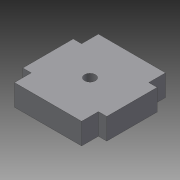
# Autodesk Inventor part: Frame_Upper_Plate_Pulley_A
Saved by Autodesk Inventor 2014 (Build 180170000, 170)
## iProperties
Created: 2014-08-25
Part Number: Frame_Upper_Plate_Pulley_A
Material: Generic
Document SubType Name: Modeling
Designer: ThatOtherGuy
Density: 1 g/cm^3
Appearance: Default
Author: ThatOtherGuy
Autodesk Inventor part; units mm, degrees
ref_plane "YZ Plane" through (0, 0, 0) normal (1, 0, 0) x (0, 1, 0)
ref_plane "XZ Plane" through (0, 0, 0) normal (0, 1, 0) x (-1, 0, 0)
ref_plane "XY Plane" through (0, 0, 0) normal (0, 0, 1) x (1, 0, 0)
sketch "Sketch1" plane through (0, 0, 0) normal (0, 0, 1) x (1, 0, 0)
  line L0 (0, 0) -> (2.5, 0)
  line L1 (2.5, 0) -> (2.5, -5)
  line L2 (2.5, -5) -> (22.5, -5)
  line L3 (22.5, -5) -> (22.5, 0)
  line L4 (22.5, 0) -> (25, 0)
  line L5 (25, 0) -> (25, 15)
  line L6 (25, 15) -> (22.5, 15)
  line L7 (22.5, 15) -> (22.5, 20)
  line L8 (22.5, 20) -> (2.5, 20)
  line L9 (2.5, 20) -> (2.5, 15)
  line L10 (2.5, 15) -> (0, 15)
  line L11 (0, 15) -> (0, 0)
  circle A0 centre (12.5, 7.5) radius 1.6
  point P0 (0, 7.5)
  point P1 (12.5, 20)
  dimension "d0" = 20
  dimension "d1" = 15
  dimension "d2" = 25
  dimension "d3" = 5
  dimension "d4" = 3.2
  constraints: 24 end point, 8 parallel, 6 equal length, 2 collinear, 2 midpoint, 1 centre point, 1 horizontal, 1 horizontal alignment, 1 perpendicular, 1 vertical alignment
  measures "d0" distance of L7.end L8.end
  measures "d1" distance of L10.end L0.start
  measures "d2" distance between parallel lines of L11 L5
  measures "d3" distance of L6.end L7.end
  measures "d4" diameter of A0
extrude "Extrusion1" add sketch "Sketch1" along normal blind 6.731
equation "\"d10\" = THICKB"
equation "\"THICKA\" = 3.175"
equation "\"THICKB\" = 6.731"
equation "\"THICKC\" = 12.7"
equation "\"BALLDIA\" = 12"
equation "\"MAGDIA\" = 9.5"
equation "\"THICKPLY\" = 5"
body "Solid1"
